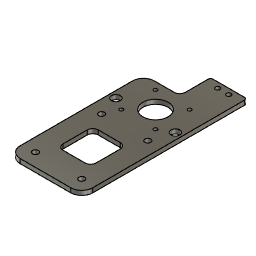
Laser Carriage - Motor Side (Autodesk Fusion 360 design; units mm, degrees)
Autodesk Fusion 360 part; units mm, degrees
sketch "Sketch1" plane through (0, 0, 0) normal (0, 0, 1) x (1, 0, 0) in component "Laser Carriage - Motor Side"
  line L0 (0, 0) -> (66, 0)
  line L1 (66, 0) -> (66, 122)
  line L2 (66, 122) -> (0, 122)
  line L3 (0, 122) -> (0, 0)
  dimension "d1" = 66
  dimension "d2" = 122
  constraint horizontal L0
  constraint vertical L1
  constraint horizontal L2
  constraint vertical L3
  constraint coincident L0.start L3.end
  measures "d1" distance of L0.start L0.end
  measures "d2" distance of L0.start L2.end
extrude "Extrude1" add sketch "Sketch1" along normal blind 4 in component "Laser Carriage - Motor Side"
sketch "Sketch2" plane through (0, 0, 4) normal (0, 0, 1) x (-1, 0, 0) in component "Laser Carriage - Motor Side"
  line L0 (0, -122) -> (0, 0)
  line L1 (0, 0) -> (-66, 0)
  line L2 (-66, 0) -> (-66, -122)
  line L3 (-66, -122) -> (0, -122)
  line L4 (-12, -122) -> (-12, 0) construction
  line L5 (-54, -122) -> (-54, 0) construction
  line L6 (0, -12) -> (-66, -12) construction
  line L7 (0, -72) -> (-66, -72) construction
  circle A0 centre (-12, -72) radius 12 construction
  circle A1 centre (-54, -72) radius 12 construction
  circle A2 centre (-12, -72) radius 2.65
  circle A3 centre (-54, -72) radius 2.65
  line L8 (-12, 0) -> (-12, -122) construction
  line L9 (-54, 0) -> (-54, -122) construction
  circle A4 centre (-12, -12) radius 12 construction
  circle A5 centre (-54, -12) radius 12 construction
  circle A6 centre (-12, -12) radius 2.65
  circle A7 centre (-54, -12) radius 2.65
  line L10 (0, -85) -> (-66, -85) construction
  line L11 (-33, -85) -> (-33, 0) construction
  line L12 (0, -42) -> (-66, -42) construction
  line L13 (-48, -58) -> (-18, -58)
  line L14 (-18, -58) -> (-18, -26)
  line L15 (-18, -26) -> (-48, -26)
  line L16 (-48, -26) -> (-48, -58)
  line L17 (-48, -58) -> (-18, -26) construction
  line L18 (-18, -58) -> (-48, -26) construction
  point P0 (-33, -42)
  dimension "d8" = 12
  dimension "d13" = 24
  dimension "d14" = 24
  dimension "d16" = 5.3
  dimension "d17" = 5.3
  dimension "d40" = 60
  dimension "d53" = 24
  dimension "d54" = 24
  dimension "d55" = 5.3
  dimension "d56" = 5.3
  dimension "d234" = 13
  dimension "d237" = 42
  dimension "d238" = 21
  dimension "d239" = 42
  dimension "d240" = 21
  dimension "d324" = 30
  constraint coincident L3 L4.start
  constraint coincident L1 L4.end
  constraint perpendicular L1 L4
  constraint coincident L3 L5.start
  constraint coincident L1 L5.end
  constraint perpendicular L1 L5
  constraint coincident L1 L11.end
  constraint coincident L0 L6.start
  constraint coincident L2 L6.end
  constraint perpendicular L2 L6
  constraint coincident L0 L7.start
  constraint coincident L2 L7.end
  constraint perpendicular L2 L7
  constraint coincident L7 A0.centre
  constraint coincident L4 A0.centre
  constraint coincident L7 A1.centre
  constraint coincident L5 A1.centre
  constraint concentric A0 A2
  constraint concentric A1 A3
  constraint perpendicular L3 L8
  constraint perpendicular L3 L9
  constraint coincident L8 A4.centre
  constraint coincident L6 A4.centre
  constraint coincident L9 A5.centre
  constraint coincident L6 A5.centre
  constraint concentric A4 A6
  constraint concentric A5 A7
  constraint coincident L0 L10.start
  constraint coincident L2 L10.end
  constraint perpendicular L2 L10
  constraint midpoint L10 L11.start
  constraint coincident L0 L12.start
  constraint coincident L2 L12.end
  constraint perpendicular L2 L12
  constraint horizontal L13
  constraint perpendicular L13 L14
  constraint parallel L13 L15
  constraint parallel L14 L16
  constraint coincident L17 P0
  constraint coincident L18 P0
  constraint midpoint L12 P0
  measures "d8" distance of L1 L6
  measures "d13" diameter of A0
  measures "d14" diameter of A1
  measures "d16" diameter of A2
  measures "d17" diameter of A3
  measures "d40" distance of L6 L7
  measures "d53" diameter of A4
  measures "d54" diameter of A5
  measures "d55" diameter of A6
  measures "d56" diameter of A7
  measures "d234" distance of A0.centre L10
  measures "d237" distance of L4 L5
  measures "d238" distance of L4 L11
  measures "d239" distance of L8 L9
  measures "d240" distance of L8 L11
  measures "d324" distance of L6 L12
extrude "Extrude2" cut sketch "Sketch2" against normal up to surface (4 mm away) contours A2 | A3 | A6 | A7 | L13 L14 L15 L16 in component "Laser Carriage - Motor Side"
sketch "Sketch16" plane through (0, 0, 4) normal (0, 0, 1) x (-1, 0, 0) in component "Laser Carriage - Motor Side"
  circle A0 centre (-54, -72) radius 2.65
  circle A1 centre (-12, -72) radius 2.65
  line L0 (-66, -122) -> (0, -122)
  line L1 (0, -122) -> (0, 0)
  line L2 (0, 0) -> (-66, 0)
  line L3 (-66, 0) -> (-66, -122)
  circle A2 centre (-12, -12) radius 2.65
  circle A3 centre (-54, -12) radius 2.65
  line L4 (0, -91) -> (-66, -91) construction
  line L5 (-66, -122) -> (0, -122) construction
  line L6 (-6, 0) -> (-6, -122) construction
  line L7 (0, -122) -> (0, 0) construction
  line L8 (-60, 0) -> (-60, -122) construction
  circle A4 centre (-6, -91) radius 4
  circle A5 centre (-60, -91) radius 4
  line L9 (0, 0) -> (-66, 0)
  line L10 (-48, -26) -> (-18, -26)
  line L11 (-18, -26) -> (-18, -58)
  line L12 (-18, -58) -> (-48, -58)
  line L13 (-48, -58) -> (-48, -26)
  dimension "d268" = 6
  dimension "d269" = 6
  dimension "d270" = 8
  dimension "d271" = 8
  dimension "d273" = 91
  constraint coincident L1 L4.start
  constraint coincident L3 L4.end
  constraint perpendicular L3 L4
  constraint coincident L5 L6.end
  constraint coincident L2 L8.start
  constraint coincident L5 L8.end
  constraint coincident L4 A4.centre
  constraint coincident L6 A4.centre
  constraint coincident L4 A5.centre
  constraint coincident L8 A5.centre
  measures "d268" distance of L6 L7
  measures "d269" distance of L3 L8
  measures "d270" diameter of A4
  measures "d271" diameter of A5
  measures "d273" distance of L2 L4
extrude "Extrude17" cut sketch "Sketch16" against normal up to surface (4 mm away) contours A4 | A5 in component "Laser Carriage - Motor Side"
sketch "Sketch18" plane through (0, 0, 4) normal (0, 0, 1) x (-1, 0, 0) in component "Laser Carriage - Motor Side"
  line L0 (-66, -122) -> (0, -122)
  line L1 (-33, -122) -> (-33, 0) construction
  line L2 (0, 0) -> (-66, 0) construction
  line L3 (-48.5, -122) -> (-48.5, 0) construction
  line L4 (-17.5, 0) -> (-17.5, -122) construction
  line L5 (-3, -115.5) -> (-63, -115.5) construction
  line L6 (-3, -84.5) -> (-63, -84.5) construction
  line L7 (-3, -100) -> (-63, -100) construction
  circle A0 centre (-33, -100) radius 11.5
  circle A1 centre (-17.5, -115.5) radius 1.65
  circle A2 centre (-48.5, -115.5) radius 1.65
  circle A3 centre (-17.5, -84.5) radius 1.65
  circle A4 centre (-48.5, -84.5) radius 1.65
  line L8 (-3, -122) -> (-63, -122) construction
  line L9 (-55, -122) -> (-11, -122) construction
  line L10 (-11, -122) -> (-11, -78) construction
  line L11 (-11, -78) -> (-55, -78) construction
  line L12 (-55, -78) -> (-55, -122) construction
  line L13 (-55, -122) -> (-11, -78) construction
  line L14 (-11, -122) -> (-55, -78) construction
  point P0 (-33, -100)
  dimension "d275" = 15.5
  dimension "d276" = 15.5
  dimension "d279" = 100
  dimension "d280" = 15.5
  dimension "d281" = 15.5
  dimension "d283" = 23
  dimension "d284" = 3.3
  dimension "d285" = 3.3
  dimension "d286" = 3.3
  dimension "d287" = 3.3
  dimension "d288" = 6.5
  dimension "d289" = 44
  dimension "d290" = 44
  constraint midpoint L0 L1.start
  constraint perpendicular L0 L1
  constraint coincident L0 L3.start
  constraint coincident L2 L3.end
  constraint perpendicular L2 L3
  constraint coincident L2 L4.start
  constraint coincident L0 L4.end
  constraint perpendicular L0 L4
  constraint horizontal L5
  constraint horizontal L6
  constraint perpendicular L3 L7
  constraint midpoint L7 P0
  constraint coincident L4 A1.centre
  constraint coincident L5 A1.centre
  constraint coincident L3 A2.centre
  constraint coincident L5 A2.centre
  constraint coincident L4 A3.centre
  constraint coincident L6 A3.centre
  constraint coincident L3 A4.centre
  constraint coincident L6 A4.centre
  constraint perpendicular L3 L8
  constraint horizontal L9
  constraint perpendicular L9 L10
  constraint parallel L9 L11
  constraint parallel L10 L12
  constraint coincident L13 P0
  constraint coincident L14 P0
  constraint coincident P0 A0.centre
  measures "d275" distance of L1 L3
  measures "d276" distance of L1 L4
  measures "d279" distance of L2 L7
  measures "d280" distance of L5 L7
  measures "d281" distance of L6 L7
  measures "d283" diameter of A0
  measures "d284" diameter of A1
  measures "d285" diameter of A2
  measures "d286" diameter of A3
  measures "d287" diameter of A4
  measures "d288" distance of L5 L8
  measures "d289" distance of L10.end L11.end
  measures "d290" distance of L9.end L10.end
extrude "Extrude18" cut sketch "Sketch18" against normal up to surface (4 mm away) in component "Laser Carriage - Motor Side"
sketch "Sketch20" plane through (0, 0, 0) normal (0, 0, -1) x (1, 0, 0) in component "Laser Carriage - Motor Side"
  circle A0 centre (17.5, -115.5) radius 1.65
  circle A1 centre (48.5, -115.5) radius 1.65
  circle A2 centre (17.5, -84.5) radius 1.65
  circle A3 centre (33, -100) radius 11.5
  circle A4 centre (48.5, -84.5) radius 1.65
  circle A5 centre (6, -91) radius 4
  circle A6 centre (60, -91) radius 4
  circle A7 centre (54, -72) radius 2.65
  circle A8 centre (12, -12) radius 2.65
  circle A9 centre (12, -72) radius 2.65
  circle A10 centre (54, -12) radius 2.65
  line L0 (0, 0) -> (0, -122)
  line L1 (0, -122) -> (66, -122)
  line L2 (66, -122) -> (66, 0)
  line L3 (66, 0) -> (0, 0)
  line L4 (66, -122) -> (66, -150)
  line L5 (33, -122) -> (33, -150)
  line L6 (33, -150) -> (66, -150)
  line L7 (18, -26) -> (48, -26)
  line L8 (48, -26) -> (48, -58)
  line L9 (48, -58) -> (18, -58)
  line L10 (18, -58) -> (18, -26)
  dimension "d303" = 28
  dimension "d304" = 28
  constraint coincident L1.end L2.start
  constraint perpendicular L1 L4
  constraint midpoint L1 L5.start
  constraint perpendicular L1 L5
  measures "d303" distance of L1.end L4.end
  measures "d304" distance of L5.start L5.end
extrude "Extrude20" add sketch "Sketch20" against normal blind 4 contours L1 L4 L5 L6 in component "Laser Carriage - Motor Side"
sketch "Sketch21" plane through (0, 0, 4) normal (0, 0, 1) x (-1, 0, 0) in component "Laser Carriage - Motor Side"
  circle A0 centre (-17.5, -115.5) radius 1.65
  circle A1 centre (-48.5, -115.5) radius 1.65
  circle A2 centre (-17.5, -84.5) radius 1.65
  circle A3 centre (-33, -100) radius 11.5
  circle A4 centre (-48.5, -84.5) radius 1.65
  circle A5 centre (-6, -91) radius 4
  circle A6 centre (-60, -91) radius 4
  line L0 (0, -122) -> (0, 0)
  line L1 (0, 0) -> (-66, 0)
  line L2 (-66, 0) -> (-66, -150)
  line L3 (-66, -150) -> (-33, -150)
  line L4 (-33, -150) -> (-33, -122)
  line L5 (-33, -122) -> (0, -122)
  circle A7 centre (-54, -72) radius 2.65
  circle A8 centre (-12, -12) radius 2.65
  circle A9 centre (-12, -72) radius 2.65
  circle A10 centre (-54, -12) radius 2.65
  line L6 (-49.5, -150) -> (-49.5, -122) construction
  line L7 (-33, -140) -> (-66, -140) construction
  line L8 (-55, -122) -> (-11, -122) construction
  line L9 (-33, -145) -> (-66, -145) construction
  line L10 (-54.5, -150) -> (-54.5, -140) construction
  line L11 (-44.5, -150) -> (-44.5, -140) construction
  circle A11 centre (-44.5, -145) radius 2.05
  circle A12 centre (-54.5, -145) radius 2.05
  line L12 (-48, -26) -> (-18, -26)
  line L13 (-18, -26) -> (-18, -58)
  line L14 (-18, -58) -> (-48, -58)
  line L15 (-48, -58) -> (-48, -26)
  dimension "d309" = 18
  dimension "d310" = 5
  dimension "d311" = 10
  dimension "d312" = 5
  dimension "d313" = 4.1
  dimension "d314" = 4.1
  constraint midpoint L3 L6.start
  constraint perpendicular L3 L6
  constraint coincident L4 L7.start
  constraint coincident L2 L7.end
  constraint perpendicular L2 L7
  constraint coincident L4 L9.start
  constraint coincident L2 L9.end
  constraint perpendicular L2 L9
  constraint coincident L3 L10.start
  constraint coincident L7 L10.end
  constraint perpendicular L7 L10
  constraint coincident L3 L11.start
  constraint coincident L7 L11.end
  constraint perpendicular L7 L11
  constraint midpoint L11 A11.centre
  constraint midpoint L10 A12.centre
  measures "d309" distance of L7 L8
  measures "d310" distance of L3 L9
  measures "d311" distance of L10 L11
  measures "d312" distance of L6 L11
  measures "d313" diameter of A11
  measures "d314" diameter of A12
extrude "Extrude21" cut sketch "Sketch21" against normal blind 4 contours A11 | A12 in component "Laser Carriage - Motor Side"
fillet "Fillet11" radius 5 1 edges at (33, 122, 2) in component "Laser Carriage - Motor Side"
fillet "Fillet11" radius 2 2 edges at (33, 150, 2) (66, 150, 2) in component "Laser Carriage - Motor Side"
fillet "Fillet11" radius 10 3 edges at (0, 122, 2) (0, 0, 2) (66, 0, 2) in component "Laser Carriage - Motor Side"
fillet "Fillet11" radius 5 4 edges at (18, 58, 2) (48, 58, 2) (48, 26, 2) (18, 26, 2) in component "Laser Carriage - Motor Side"
component "Laser Carriage - Motor Side" placed x (1, 0, 0) y (0, 1, 0) z (0, 0, 1) at (0, 0, 0)
named bodies: "Laser Carriage - Motor Side"
